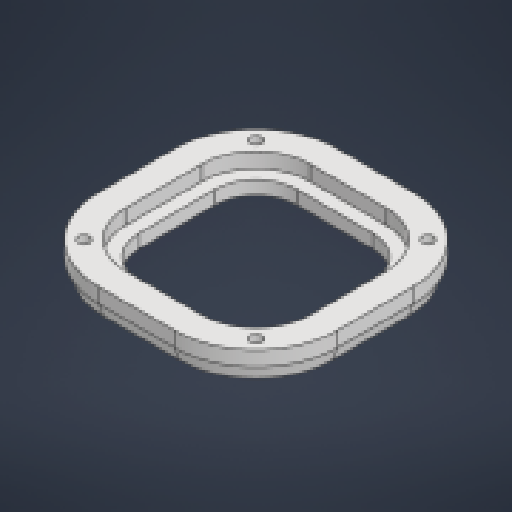
# Autodesk Inventor part: subcap
Saved by Autodesk Inventor 2024 (Build 280153000, 153)
## iProperties
Created: 2024-06-29
Part Number: subcap
Material: Generic
Document SubType Name: Modeling
Designer: markm
Density: 1 g/cm^3
Appearance: Default
Author: markm
Autodesk Inventor part; units mm, degrees
ref_plane "YZ Plane" through (0, 0, 0) normal (1, 0, 0) x (0, 1, 0)
ref_plane "XZ Plane" through (0, 0, 0) normal (0, 1, 0) x (-1, 0, 0)
ref_plane "XY Plane" through (0, 0, 0) normal (0, 0, 1) x (1, 0, 0)
sketch "Sketch1" plane through (0, 0, 0) normal (0, 1, 0) x (-1, 0, 0)
  line L0 (-7, 17) -> (7, 17)
  line L1 (17, 7) -> (17, -7)
  line L2 (7, -17) -> (-7, -17)
  line L3 (-17, -7) -> (-17, 7)
  line L4 (-17, 17) -> (17, -17) construction
  line L5 (17, 17) -> (-17, -17) construction
  arc A0 (17, 7) -> (7, 17) centre (7, 7) ccw
  arc A1 (7, -17) -> (17, -7) centre (7, -7) ccw
  arc A2 (-17, -7) -> (-7, -17) centre (-7, -7) ccw
  arc A3 (-7, 17) -> (-17, 7) centre (-7, 7) ccw
  line L6 (-7, -22) -> (7, -22)
  arc A4 (7, -22) -> (22, -7) centre (7, -7) ccw
  line L7 (22, -7) -> (22, 7)
  arc A5 (22, 7) -> (7, 22) centre (7, 7) ccw
  line L8 (7, 22) -> (-7, 22)
  arc A6 (-7, 22) -> (-22, 7) centre (-7, 7) ccw
  line L9 (-22, 7) -> (-22, -7)
  arc A7 (-22, -7) -> (-7, -22) centre (-7, -7) ccw
  circle A8 centre (-15.8388, -15.8388) radius 1.05
  line L10 (-14.0711, -14.0711) -> (-17.6066, -17.6066) construction
  circle A9 centre (15.8388, -15.8388) radius 1.05
  circle A10 centre (15.8388, 15.8388) radius 1.05
  circle A11 centre (-15.8388, 15.8388) radius 1.05
  line L11 (14.5, -7) -> (14.5, 7)
  arc A12 (14.5, 7) -> (7, 14.5) centre (7, 7) ccw
  line L12 (7, 14.5) -> (-7, 14.5)
  arc A13 (-7, 14.5) -> (-14.5, 7) centre (-7, 7) ccw
  line L13 (-14.5, 7) -> (-14.5, -7)
  arc A14 (-14.5, -7) -> (-7, -14.5) centre (-7, -7) ccw
  line L14 (-7, -14.5) -> (7, -14.5)
  arc A15 (7, -14.5) -> (14.5, -7) centre (7, -7) ccw
  point P0 (0, 0)
  dimension "d0" = 34
  dimension "d1" = 34
  dimension "d2" = 10
  dimension "d3" = 5
  dimension "d4" = 2.1
  dimension "d7" = 360
  dimension "d11" = 2.5
  constraints: 30 end point, 26 point on circle, 16 centre point, 8 point on line, 8 tangent, 6 parallel, 3 equal radius, 3 midpoint, 3 perpendicular, 1 horizontal, 23 other
  measures "d0" distance of L4.end L5.end
  measures "d1" distance of L5.start L4.end
  measures "d2" radius of A0
  measures "d3" radial gap between concentric circles of A2 A7
  measures "d4" diameter of A8
  measures "d11" distance between parallel lines of L1 L11
extrude "Extrusion1" add sketch "Sketch1" along normal blind 2.75 contours A7 L9 A6 L8 A5 L7 A4 L6
extrude "Extrusion2" add sketch "Sketch1" against normal blind 2.5 contours L0 A0 L1 A1 L2 A2 L3 A3 | A7 L9 A6 L8 A5 L7 A4 L6
chamfer "Chamfer1" distance 1 distance2 2.5 8 edges at (17.6066, -2.5, 17.6066) (0, -2.5, 22) (-17.6066, -2.5, 17.6066) (-22, -2.5, 0) (-17.6066, -2.5, -17.6066) (0, -2.5, -22) (17.6066, -2.5, -17.6066) (22, -2.5, 0) measured on face at (19.5, -2.5, 2.3333)
body "Solid1"
